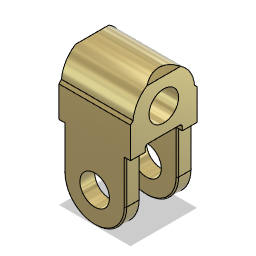
0.885.7216 - Pièce intermédiaire - IGTE 21485_232834 (Autodesk Fusion 360 design; units mm, degrees)
Autodesk Fusion 360 part; units mm, degrees
sketch "Sketch1" plane through (0, 0, 0) normal (0, 0, 1) x (1, 0, 0)
  line L0 (0, 0) -> (0, 55) construction
  line L1 (0, 12.5) -> (12.5, 12.5) construction
  arc A0 (0, 0) -> (12.5, 12.5) centre (0, 12.5) ccw
  line L2 (0, 55) -> (12.5, 55)
  line L3 (12.5, 55) -> (12.5, 12.5)
  line L4 (0, 55) -> (-12.5, 55)
  line L5 (-12.5, 55) -> (-12.5, 12.5)
  arc A1 (-12.5, 12.5) -> (0, 0) centre (0, 12.5) ccw
  line L6 (14.5, 55) -> (14.5, 12.5) construction
  line L7 (12.5, 55) -> (14.5, 53)
  line L8 (12.5, 55) -> (26.8265, 55) construction
  line L9 (14.5, 53) -> (14.5, 30)
  line L10 (14.5, 30) -> (12.5, 30)
  line L11 (-14.5, 30) -> (-12.5, 30)
  line L12 (-12.5, 55) -> (-26.8265, 55) construction
  line L13 (-14.5, 53) -> (-14.5, 30)
  line L14 (-14.5, 55) -> (-12.5, 55)
  line L15 (12.5, 55) -> (14.5, 55)
  line L16 (-12.5, 55) -> (-14.5, 53)
  dimension "d1" = 55
  dimension "d2" = 25
  dimension "d4" = 12.5
  dimension "d5" = 2
  dimension "d6" = 45
  dimension "d7" = 25
  constraint coincident L0.start A0.start
  constraint coincident L1.start A0.centre
  constraint perpendicular L0 L1
  constraint tangent A0 L3
  constraint symmetric A0.start L0 A1.end
  constraint symmetric L2.start L0 L4.start
  constraint symmetric L0 L1.end L5.end
  constraint symmetric L0 A0 A1
  constraint symmetric L0 L2.end L4.end
  constraint horizontal L8
  constraint coincident L6 L7.end
  constraint coincident L3 L10.end
  constraint perpendicular L3 L10
  constraint symmetric L0 L6.start L14.start
  constraint symmetric L0 L8.end L12.end
  constraint symmetric L0 L9.end L11.start
  constraint symmetric L0 L10.end L11.end
  constraint perpendicular L5 L14
  constraint symmetric L0 L7.end L13.start
  measures "d1" distance of L0.start L0.end
  measures "d2" diameter of A0
  measures "d4" distance of L0.end L2.end
  measures "d6" angle of L7 L8
  measures "d7" distance of L6.start L9.end
extrude "Extrude1" add sketch "Sketch1" along normal mid plane 27
sketch "Sketch2" plane through (0, 0, 13.5) normal (0, 0, 1) x (1, 0, 0)
  line L0 (12.5, 55) -> (-12.5, 55)
  line L1 (-12.5, 55) -> (-14.5, 53)
  line L2 (-14.5, 53) -> (-14.5, 30)
  line L3 (-14.5, 30) -> (-12.5, 30)
  line L4 (-12.5, 30) -> (-12.5, 12.5)
  arc A0 (-12.5, 12.5) -> (12.5, 12.5) centre (0, 12.5) ccw
  line L5 (12.5, 12.5) -> (12.5, 30)
  line L6 (12.5, 30) -> (14.5, 30)
  line L7 (14.5, 30) -> (14.5, 53)
  line L8 (14.5, 53) -> (12.5, 55)
  arc A1 (-12.5, 12.5) -> (12.5, 12.5) centre (0, 12.5) ccw
  circle A2 centre (0, 12.5) radius 6
  dimension "d10" = 12
  constraint concentric A0 A2
  measures "d10" diameter of A2
extrude "Extrude2" cut sketch "Sketch2" against normal through all contours A2
sketch "Sketch3" plane through (0, 0, 0) normal (1, 0, 0) x (0, 0, -1)
  line L0 (13.5, 18.5) -> (13.5, 6.5) construction
  line L1 (-13.5, 6.5) -> (-13.5, 18.5) construction
  line L2 (13.5, 55) -> (-13.5, 55) construction
  line L3 (13.5, 30) -> (13.5, 53) construction
  line L4 (13.5, 53) -> (13.5, 55) construction
  line L5 (-13.5, 55) -> (-13.5, 53) construction
  line L6 (-13.5, 53) -> (-13.5, 30) construction
  line L7 (-13.5, 30) -> (-13.5, 12.5) construction
  line L8 (13.5, 12.5) -> (13.5, 30) construction
  line L9 (13.5, 0) -> (13.5, 12.5) construction
  line L10 (-13.5, 12.5) -> (-13.5, 0) construction
  line L11 (13.5, 12.5) -> (-13.5, 12.5) construction
  line L12 (-13.5, 12.5) -> (-13.5, 0) construction
  line L13 (-13.5, 12.5) -> (13.5, 12.5) construction
  line L14 (13.5, 0) -> (13.5, 12.5) construction
  line L15 (13.5, 0) -> (-13.5, 0) construction
  line L16 (-13.5, 42.5) -> (13.5, 42.5) construction
  line L17 (13.5, 32.5) -> (-13.5, 32.5) construction
  line L18 (13.5, 32.5) -> (13.5, 2)
  line L19 (7.5, 31.5) -> (7.5, 0)
  line L20 (11.5, 0) -> (7.5, 0)
  line L21 (0, 32.5) -> (6.5, 32.5)
  arc A0 (7.5, 31.5) -> (6.5, 32.5) centre (6.5, 31.5) ccw
  line L22 (0, 55) -> (0, 0) construction
  circle A1 centre (0, 42.5) radius 12.5 construction
  line L23 (13.5, 42.5) -> (12.4564, 43.5436)
  line L24 (13.5, 42.5) -> (21.4057, 42.5) construction
  arc A2 (12.4564, 43.5436) -> (0, 55) centre (0, 42.5) ccw
  line L25 (13.5, 42.5) -> (13.5, 32.5)
  arc A3 (0, 55) -> (-12.4564, 43.5436) centre (0, 42.5) ccw
  line L26 (-13.5, 42.5) -> (-12.4564, 43.5436)
  line L27 (-13.5, 42.5) -> (-13.5, 32.5)
  line L28 (-13.5, 32.5) -> (-13.5, 2)
  line L29 (-11.5, 0) -> (-7.5, 0)
  line L30 (-7.5, 31.5) -> (-7.5, 0)
  arc A4 (-6.5, 32.5) -> (-7.5, 31.5) centre (-6.5, 31.5) ccw
  line L31 (0, 32.5) -> (-6.5, 32.5)
  line L32 (7.5, 0) -> (-7.5, 0)
  line L33 (-11.5, 0) -> (-13.5, 0)
  line L34 (-13.5, 2) -> (-13.5, 0)
  line L35 (13.5, 2) -> (13.5, 0)
  line L36 (13.5, 0) -> (11.5, 0)
  line L37 (13.5, 55) -> (13.5, 42.5)
  line L38 (13.5, 55) -> (0, 55)
  line L39 (0, 55) -> (-13.5, 55)
  line L40 (-13.5, 55) -> (-13.5, 42.5)
  circle A5 centre (0, 42.5) radius 6
  dimension "d12" = 30
  dimension "d13" = 20
  dimension "d16" = 1
  dimension "d17" = 25
  dimension "d18" = 135
  dimension "d21" = 12
  constraint coincident L9.start L14.start
  constraint coincident L10.end L12.end
  constraint perpendicular L15 L18
  constraint perpendicular L9 L20
  constraint parallel L18 L19
  constraint midpoint L17 L21.start
  constraint perpendicular L19 L21
  constraint tangent L19 A0
  constraint tangent L21 A0
  constraint midpoint L2 L22.start
  constraint coincident L22.end origin
  constraint midpoint L16 A1.centre
  constraint horizontal L24
  constraint coincident A1 L23.end
  constraint concentric A1 A2
  constraint tangent L2 A2
  constraint perpendicular L17 L25
  constraint symmetric L16.end L22 L16.start
  constraint symmetric L17.start L22 L17.end
  constraint symmetric L19.end L22 L29.end
  constraint symmetric L20.start L22 L29.start
  constraint symmetric L18.end L22 L28.end
  constraint symmetric L21.start L22 L31.start
  constraint symmetric L19.start L22 L30.start
  constraint symmetric L21.end L22 A4.start
  constraint symmetric A0 L22 A4
  constraint symmetric A2.end L22 A3.start
  constraint symmetric L22 L23.end A3.end
  constraint symmetric L22 A2 A3
  constraint coincident L2.start L4.end
  constraint perpendicular L24 L37
  constraint coincident L2.end L5.start
  constraint perpendicular L16 L40
  constraint concentric A3 A5
  measures "d16" radius of A0
  measures "d17" diameter of A1
  measures "d18" angle of L23 L24
  measures "d21" diameter of A5
extrude "Extrude3" cut sketch "Sketch3" along normal through all and the other way through all contours L23 A2 L37 L38 | A3 L26 L39 L40 | L19 L21 A0 L30 A4 L31 L32 | A5
fillet "Fillet1" radius 0.5 12 edges at (12.5, 21.25, -13.5) (0, 0, -13.5) (-12.5, 21.25, -13.5) (12.5, 21.25, -7.5) (0, 0, -7.5) (-12.5, 21.25, -7.5) (-12.5, 21.25, 7.5) (0, 0, 7.5) (12.5, 21.25, 7.5) (-12.5, 21.25, 13.5) (0, 0, 13.5) (12.5, 21.25, 13.5)
equation "d1 = 12.5 mm + 30 mm + 12.5 mm"
equation "d2 = ( 12.5 * 2 ) * 1 mm"
equation "d8 = 6 mm + 15 mm + 6 mm"
equation "d17 = ( 12.5 * 2 ) * 1 mm"
